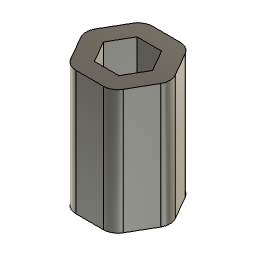
ESD_all (Autodesk Fusion 360 archive; units mm, degrees)
design "ESD_bit_holder_rev1"
Autodesk Fusion 360 part; units mm, degrees
sketch "Sketch1" plane through (0, 0, 0) normal (0, 0, 1) x (1, 0, 0)
  line L0 (-1.2861, 2.2276) -> (-2.5722, 0)
  line L1 (-2.5722, 0) -> (-1.2861, -2.2276)
  line L2 (-1.2861, -2.2276) -> (1.2861, -2.2276)
  line L3 (1.2861, -2.2276) -> (2.5722, 0)
  line L4 (2.5722, 0) -> (1.2861, 2.2276)
  line L5 (1.2861, 2.2276) -> (-1.2861, 2.2276)
  line L6 (-2.3094, 4) -> (-4.6188, 0)
  line L7 (-4.6188, 0) -> (-2.3094, -4)
  line L8 (-2.3094, -4) -> (2.3094, -4)
  line L9 (2.3094, -4) -> (4.6188, 0)
  line L10 (4.6188, 0) -> (2.3094, 4)
  line L11 (2.3094, 4) -> (-2.3094, 4)
extrude "Extrude1" add sketch "Sketch1" along normal blind 13
extrude "Extrude2" add sketch "Sketch1" along normal blind 1 contours L0 L1 L2 L3 L4 L5
chamfer "Chamfer1" distance 0.5 angle 45 6 edges at (1.9291, -1.1138, 1) (1.9291, 1.1138, 1) (0, 2.2276, 1) (-1.9291, 1.1138, 1) (-1.9291, -1.1138, 1) (0, -2.2276, 1)
fillet "Fillet1" radius 1.5 6 edges at (2.3094, 4, 6.5) (-2.3094, 4, 6.5) (-4.6188, 0, 6.5) (-2.3094, -4, 6.5) (2.3094, -4, 6.5) (4.6188, 0, 6.5)
